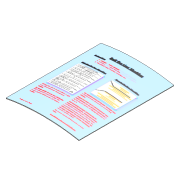
# Autodesk Inventor part: Instruction Poster
Saved by Autodesk Inventor 2018.1 (Build 221171000, 171)
## iProperties
Created: 2019-03-29
Part Number: Instruction Poster
Material: Generic
Document SubType Name: Modeling
Designer: James
Density: 1 g/cm^3
Appearance: Default
Author: James
Autodesk Inventor part; units mm, degrees
ref_plane "YZ Plane" through (0, 0, 0) normal (1, 0, 0) x (0, 1, 0)
ref_plane "XZ Plane" through (0, 0, 0) normal (0, 1, 0) x (-1, 0, 0)
sketch "Sketch1" plane through (0, 0, 0) normal (0, 1, 0) x (-1, 0, 0)
  arc A0 (114.25, 601.2412) -> (-114.25, 601.2412) centre (0, 0) ccw
  arc A1 (113.8766, 599.2763) -> (-113.8766, 599.2763) centre (0, 0) ccw
  line L0 (114.25, 601.2412) -> (113.8766, 599.2763)
  line L1 (114.25, 601.2412) -> (0, 0) construction
  line L2 (-114.25, 601.2412) -> (0, 0) construction
  line L3 (-114.25, 601.2412) -> (-113.8766, 599.2763)
  dimension "d0" = 2
  dimension "d1" = 610
  dimension "d5" = 114.25
  dimension "d6" = 228.5
  constraints: 8 end point, 4 point on circle, 2 centre point, 2 coincident, 2 collinear
  measures "d0" radial gap between concentric circles of A0 A1
  measures "d1" radius of A1
  measures "d5" horizontal distance of point (0, 0) L2.start
  measures "d6" distance of L2.start L0.start
extrude "Extrusion1" add sketch "Sketch1" along normal blind 297
ref_plane "Work Plane1" through (0, 0, 612) normal (0, 0, 1) x (1, 0, 0)
sketch "Sketch2" plane through (0, 0, 612) normal (0, 0, 1) x (1, 0, 0)
  line L0 (-114.25, 297) -> (115.5379, 297) construction
  line L1 (115.5379, 297) -> (115.5379, 0) construction
  line L2 (115.5379, 0) -> (-114.25, 0) construction
  line L3 (-114.25, 0) -> (-114.25, 297) construction
  point P0 (0, 0)
  point P1 (114.25, 0)
  constraints: 1 coincident, 1 horizontal alignment, 1 vertical alignment, 2 other
decal "Decal1"
equation "\"d5\" = 0.5 * d6"
body "Solid1"
